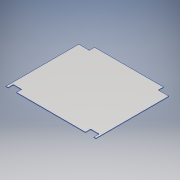
# Autodesk Inventor part: BK-BKT120-BasePlate-Short
Saved by Autodesk Inventor 2017 (Build 210142000, 142)
## iProperties
Created: 2016-09-24
Part Number: BK-BKT120-BasePlate-Short
Material: Aluminum 6061
Document SubType Name: Modeling
Designer: vslabsal
Density: 2.7 g/cm^3
Appearance: Aluminum - Flat
Author: vslabsal
Autodesk Inventor part; units mm, degrees
ref_plane "YZ Plane" through (0, 0, 0) normal (1, 0, 0) x (0, 1, 0)
ref_plane "XZ Plane" through (0, 0, 0) normal (0, 1, 0) x (-1, 0, 0)
ref_plane "XY Plane" through (0, 0, 0) normal (0, 0, 1) x (1, 0, 0)
sketch "Sketch1" plane through (0, 0, 0) normal (0, 0, 1) x (1, 0, 0)
  line L0 (270.51, 284.48) -> (-270.51, -284.48) construction
  line L1 (-270.51, 284.48) -> (270.51, -284.48) construction
  line L2 (207.005, 234.48) -> (-207.015, 234.48)
  line L3 (-210.185, 203.2) -> (-270.51, 203.2)
  arc A0 (-210.185, 203.2) -> (-207.015, 206.375) centre (-210.19, 206.375) ccw
  line L4 (207.005, 234.48) -> (207.005, 206.375)
  line L5 (270.51, 203.2) -> (210.185, 203.2)
  arc A1 (207.005, 206.375) -> (210.185, 203.2) centre (210.18, 206.375) ccw
  line L6 (-257.81, -234.48) -> (-257.81, -206.375)
  line L7 (-207.01, -234.48) -> (-207.01, -206.375)
  arc A2 (-254.635, -203.2) -> (-257.81, -206.375) centre (-254.635, -206.375) ccw
  arc A3 (-207.01, -206.375) -> (-210.185, -203.2) centre (-210.185, -206.375) ccw
  line L8 (-254.635, -203.2) -> (-210.185, -203.2)
  line L9 (207.01, -234.48) -> (207.01, -206.375)
  line L10 (257.81, -234.48) -> (257.81, -206.375)
  arc A4 (210.185, -203.2) -> (207.01, -206.375) centre (210.185, -206.375) ccw
  arc A5 (257.81, -206.375) -> (254.635, -203.2) centre (254.635, -206.375) ccw
  line L11 (210.185, -203.2) -> (254.635, -203.2)
  line L12 (270.51, 203.2) -> (270.51, -234.48)
  line L13 (257.81, -234.48) -> (270.51, -234.48)
  line L14 (-270.51, 203.2) -> (-270.51, -234.48)
  line L15 (-270.51, -234.48) -> (-257.81, -234.48)
  line L16 (-207.01, -234.48) -> (207.01, -234.48)
  line L17 (-207.015, 234.48) -> (-207.015, 206.375)
  point P0 (0, 0)
  point P1 (0, 0)
  point P2 (-207.015, 206.375)
  dimension "d14" = 414.02
  dimension "d20" = 60.325
  dimension "d22" = 28.105
  dimension "d23" = 60.325
  dimension "d28" = 44.45
  dimension "d29" = 50.8
  dimension "d34" = 437.68
  dimension "d38" = 437.68
  constraints: 36 end point, 18 point on circle, 8 vertical, 7 horizontal, 6 centre point, 2 midpoint, 2 tangent, 1 perpendicular, 1 point on line
  measures "d14" distance of L2.end L2.start
  measures "d20" distance of L3.start L3.end
  measures "d22" distance of L2.start L4.end
  measures "d23" distance of L5.start L5.end
  measures "d28" distance of L8.start L8.end
  measures "d29" distance between parallel lines of L7 L6
  measures "d34" distance of L5.start L12.end
  measures "d38" distance of L3.end L14.end
extrude "Extrusion1" add sketch "Sketch1" along normal blind 3.175
body "Solid1"
